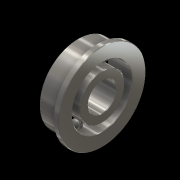
# Autodesk Inventor part: F608 - 8 x 22 x 7
Saved by Autodesk Inventor 2016 (Build 200138000, 138)
## iProperties
Created: 2019-09-20
Part Number: F608 - 8 x 22 x 7
Material: Generic
Document SubType Name: Modeling
Designer: xyz-150G
Density: 1 g/cm^3
Appearance: Steel - Polished
Mass: 1.81571 g
Surface Area: 20.7306 cm^2
Volume: 1.81571 cm^3
Author: xyz-150G
Autodesk Inventor part; units mm, degrees
ref_plane "YZ Plane" through (0, 0, 0) normal (1, 0, 0) x (0, 1, 0)
ref_plane "XZ Plane" through (0, 0, 0) normal (0, 1, 0) x (-1, 0, 0)
ref_plane "XY Plane" through (0, 0, 0) normal (0, 0, 1) x (1, 0, 0)
sketch "Sketch2" plane through (0, 0, 0) normal (0, 0, 1) x (1, 0, 0)
  line L0 (-6.85, 4) -> (-0.15, 4)
  line L1 (0, 4.15) -> (0, 6.2833)
  line L2 (-0.15, 6.4333) -> (-6.85, 6.4333)
  line L3 (-7, 6.2833) -> (-7, 4.15)
  line L4 (-6.85, 11) -> (-1.6061, 11)
  line L5 (-0.15, 8.5667) -> (-6.85, 8.5667)
  line L6 (-7, 8.7167) -> (-7, 10.85)
  line L7 (-1.5, 11) -> (-1.5, 11.1061) construction
  line L8 (-1.35, 12.5) -> (-0.15, 12.5)
  line L9 (-2.3, 0) -> (0, 0)
  line L10 (-7, 6.4333) -> (-7, 8.5667) construction
  line L11 (0, 0) -> (0, 4) construction
  line L12 (0, 8.7167) -> (0, 12.35)
  line L13 (-1.6061, 11) -> (-1.5, 10.8939)
  line L14 (-1.6061, 11) -> (-1.4561, 11) construction
  line L15 (-1.5, 10.8939) -> (-1.3939, 11)
  line L16 (-1.3939, 11) -> (-1.5, 11.1061)
  line L17 (-1.447, 10.947) -> (-1.5, 11) construction
  line L18 (-1.5, 11.1061) -> (-1.5, 12.35)
  line L19 (-1.6061, 11) -> (-1.5, 11) construction
  line L20 (-7, 10.85) -> (-6.85, 11)
  line L21 (-7, 8.7167) -> (-6.85, 8.5667)
  line L22 (-6.85, 6.4333) -> (-7, 6.2833)
  line L23 (-7, 4.15) -> (-6.85, 4)
  line L24 (-0.15, 4) -> (0, 4.15)
  line L25 (0, 6.2833) -> (-0.15, 6.4333)
  line L26 (-0.15, 8.5667) -> (0, 8.7167)
  line L27 (0, 12.35) -> (-0.15, 12.5)
  line L28 (-1.35, 12.5) -> (-1.5, 12.35)
  point P0 (0, 0)
  point P1 (-7, 4)
  point P2 (0, 6.4333)
  point P3 (-7, 11)
  point P4 (0, 8.5667)
  point P5 (-1.5, 12.5)
  point P6 (0, 12.5)
  dimension "d" = 8
  dimension "D" = 22
  dimension "C2" = 1.5
  dimension "d5" = 45
  dimension "d6" = 0.15
  dimension "D2" = 25
  dimension "d8" = 0.15
  dimension "d9" = 0.15
  dimension "d10" = 0.15
  dimension "d11" = 0.15
  dimension "d12" = 0.15
  dimension "d13" = 0.15
  dimension "d14" = 0.15
  dimension "d15" = 0.15
  dimension "d16" = 0.15
  dimension "d17" = 0.15
  dimension "d18" = 0.15
  dimension "d19" = 0.15
  dimension "d20" = 0.15
  dimension "d21" = 0.15
  dimension "d22" = 0.15
  dimension "d23" = 0.15
  dimension "d24" = 0.15
  dimension "d25" = 0.15
  dimension "bd" = 2.1333
  dimension "B1" = 7
  constraints: 58 end point, 20 point on line, 6 parallel, 5 horizontal, 4 equal length, 4 perpendicular, 3 vertical, 1 coincident, 1 collinear, 1 midpoint
  measures "d" diameter of L0 L9
  measures "D" diameter of L4 L9
  measures "C2" distance of point (-1.5, 12.5) point (0, 12.5)
  measures "d5" angle of L13 L14
  measures "d6" distance of L13.end L15.end
  measures "D2" diameter of L8 L9
  measures "d8" distance of L6.end point (-7, 11)
  measures "d9" distance of L4.start point (-7, 11)
  measures "d10" distance of L6.start L10.end
  measures "d11" distance of L5.end L10.end
  measures "d12" distance of L2.end L10.start
  measures "d13" distance of L3.start L10.start
  measures "d14" distance of L3.end point (-7, 4)
  measures "d15" distance of L0.start point (-7, 4)
  measures "d16" distance of L0.end L11.end
  measures "d17" distance of L1.start L11.end
  measures "d18" distance of L1.end point (0, 6.433)
  measures "d19" distance of L2.start point (0, 6.433)
  measures "d20" distance of L5.start point (0, 8.567)
  measures "d21" distance of L12.start point (0, 8.567)
  measures "d22" distance of L12.end point (0, 12.5)
  measures "d23" distance of L8.end point (0, 12.5)
  measures "d24" distance of L8.start point (-1.5, 12.5)
  measures "d25" distance of L18.end point (-1.5, 12.5)
  measures "bd" distance between parallel lines of L2 L5
  measures "B1" distance between parallel lines of L12 L6
revolve "Revolution1" add sketch "Sketch2" angle 360 about axis through (-2.3, 0, 0) along (1, 0, 0)
sketch "Sketch3" plane through (0, 0, 0) normal (0, 0, 1) x (1, 0, 0)
  line L0 (-0.15, 8.5667) -> (-6.85, 8.5667) construction
  line L1 (-6.85, 6.4333) -> (-0.15, 6.4333) construction
  line L2 (-3.5, 8.5667) -> (-3.5, 6.4333)
  arc A0 (-3.5, 6.22) -> (-3.5, 8.78) centre (-3.5, 7.5) ccw construction
  line L3 (-3.5, 8.5667) -> (-3.5, 8.78)
  line L4 (-3.5, 6.4333) -> (-3.5, 6.22)
  arc A1 (-4.2075, 6.4333) -> (-3.5, 6.22) centre (-3.5, 7.5) ccw
  arc A2 (-3.5, 8.78) -> (-4.2075, 6.4333) centre (-3.5, 7.5) ccw
  point P0 (0, 0)
  dimension "d28" = 2.56
  constraints: 6 end point, 6 point on circle, 3 centre point, 3 midpoint, 2 point on line, 1 perpendicular, 1 vertical
  measures "d28" diameter of A0
revolve "Revolution2" add sketch "Sketch3" angle 360 about axis through (-3.5, 8.5667, 0) along (0, -1, 0)
pattern_circular "Circular Pattern1" count 6 over 360 about axis through (-10, 0, 0) along (1, 0, 0) of "Revolution2"
equation "\"d6\" = 0.1 * C2"
equation "\"d8\" = 0.1 * C2"
equation "\"d9\" = d8"
equation "\"d10\" = d8"
equation "\"d11\" = d10"
equation "\"d12\" = d8"
equation "\"d13\" = d12"
equation "\"d14\" = d8"
equation "\"d15\" = d14"
equation "\"d16\" = d8"
equation "\"d17\" = d16"
equation "\"d18\" = d8"
equation "\"d19\" = d18"
equation "\"d20\" = d8"
equation "\"d21\" = d20"
equation "\"d22\" = d8"
equation "\"d23\" = d22"
equation "\"d24\" = d8"
equation "\"d25\" = d24"
equation "\"d28\" = 1.2 * bd"
body "Solid1"
